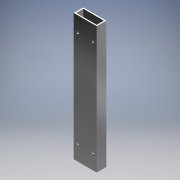
# Autodesk Inventor part: Middle Bar
Saved by Autodesk Inventor 2019.4 (Build 234330000, 330)
## iProperties
Created: 2020-01-10
Part Number: Middle Bar
Material: Aluminum 6061
Document SubType Name: Modeling
Designer: Mark
Mass: 424.894 g
Surface Area: 1058.6 cm^2
Volume: 157.368 cm^3
Density: 2.7 g/cm^3
Appearance: Aluminum - Flat
Author: Mark
Autodesk Inventor part; units mm, degrees
ref_plane "YZ Plane" through (0, 0, 0) normal (1, 0, 0) x (0, 1, 0)
ref_plane "XZ Plane" through (0, 0, 0) normal (0, 1, 0) x (-1, 0, 0)
ref_plane "XY Plane" through (0, 0, 0) normal (0, 0, 1) x (1, 0, 0)
sketch "Sketch1" plane through (0, 0, 0) normal (0, 1, 0) x (-1, 0, 0)
  line L0 (-30, 12.5) -> (30, 12.5)
  line L1 (30, 12.5) -> (30, -12.5)
  line L2 (30, -12.5) -> (-30, -12.5)
  line L3 (-30, -12.5) -> (-30, 12.5)
  line L4 (-30, 12.5) -> (30, -12.5) construction
  line L5 (30, 12.5) -> (-30, -12.5) construction
  line L6 (-27, 9.5) -> (27, 9.5)
  line L7 (27, 9.5) -> (27, -9.5)
  line L8 (27, -9.5) -> (-27, -9.5)
  line L9 (-27, -9.5) -> (-27, 9.5)
  line L10 (-27, 9.5) -> (27, -9.5) construction
  line L11 (27, 9.5) -> (-27, -9.5) construction
  point P0 (0, 0)
  dimension "d0" = 60
  dimension "d1" = 25
  dimension "d2" = 54
  dimension "d3" = 19
  constraints: 24 end point, 4 midpoint, 4 parallel, 2 horizontal, 2 perpendicular
  measures "d0" distance of L1.end L2.end
  measures "d1" distance of L0.end L1.end
  measures "d2" distance of L7.end L8.end
  measures "d3" distance of L6.end L7.end
extrude "Extrusion1" add sketch "Sketch1" along normal blind 332.5
sketch "Sketch2" plane through (30, 0, -12.5) normal (0, 0, -1) x (-1, 0, 0)
  circle A0 centre (50, 40) radius 2.75
  circle A1 centre (10, 40) radius 2.75
  line L0 (60, 0) -> (0, 0) projected
  line L1 (60, 0) -> (60, 332.5) projected
  line L2 (0, 0) -> (0, 332.5) projected
  circle A2 centre (10, 292.5) radius 2.75
  circle A3 centre (50, 292.5) radius 2.75
  line L3 (0, 332.5) -> (60, 332.5) projected
  point P0 (30, 0)
  dimension "d6" = 5.5
  dimension "d7" = 5.5
  dimension "d8" = 40
  dimension "d9" = 10
  dimension "d10" = 10
  dimension "d11" = 40
  dimension "d12" = 5.5
  dimension "d13" = 5.5
  dimension "d14" = 40
  dimension "d15" = 10
  dimension "d16" = 10
  dimension "d17" = 40
  constraints: 4 centre point
  measures "d6" diameter of A0
  measures "d7" diameter of A1
  measures "d8" distance from line of L0 A1.centre
  measures "d9" distance from line of L1 A0.centre
  measures "d10" distance from line of L2 A1.centre
  measures "d11" distance from line of L0 A0.centre
  measures "d12" diameter of A2
  measures "d13" diameter of A3
  measures "d14" distance from line of L3 A3.centre
  measures "d15" distance from line of L1 A3.centre
  measures "d16" distance from line of L2 A2.centre
  measures "d17" distance from line of L3 A2.centre
extrude "Extrusion2" cut sketch "Sketch2" against normal up to surface (25 mm away) contours A0 | A1 | A2 | A3
equation "\"d18\" = d9"
body "Solid1"
